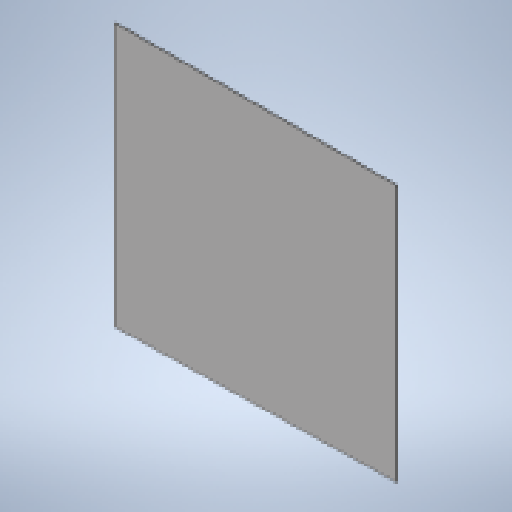
# Autodesk Inventor part: GBK 2311 shield 7
Saved by Autodesk Inventor 2026 (Build 300175000, 175)
## iProperties
Created: 2026-04-17
Part Number: GBK 2311 shield 7
Material: Steel
Document SubType Name: Sheet Metal
Designer: pokla
Stock Number: 2317
Mass: 69243.3 g
Surface Area: 44341.6 cm^2
Volume: 8820.8 cm^3
Density: 7.85 g/cm^3
Flat Pattern Width: 148 cm
Flat Pattern Length: 138.1 cm
Flat Pattern Area: 20438.8 cm^2
Sheet Metal Rule: По умолчанию_мм
Sheet Metal Width: 1480,000 мм
Sheet Metal Length: 1381,000 мм
Sheet Metal Area: 2043880,000 мм^2
Appearance: Default
Author: admin
Autodesk Inventor part; units mm, degrees
ref_plane "YZ Plane" through (0, 0, 0) normal (1, 0, 0) x (0, 1, 0)
ref_plane "XZ Plane" through (0, 0, 0) normal (0, 1, 0) x (-1, 0, 0)
ref_plane "XY Plane" through (0, 0, 0) normal (0, 0, 1) x (1, 0, 0)
sketch "Sketch1" plane through (0, 0, 0) normal (0, 0, 1) x (1, 0, 0)
  line L0 (740, -745) -> (-740, -745)
  line L1 (-740, -745) -> (-740, 745)
  line L2 (-740, 745) -> (740, 745)
  line L3 (740, 745) -> (740, -745)
  line L4 (740, -745) -> (-740, 745) construction
  line L5 (-740, -745) -> (740, 745) construction
  line L6 (-740, -636) -> (740, -602.4141)
  point P0 (0, 0)
  dimension "d0" = 1480
  dimension "d1" = 1490
  dimension "d4" = 1.3
  dimension "d9" = 1381
  dimension "d10" = 109
  measures "d0" distance of L1.end L2.end
  measures "d1" distance of L0.end L1.end
  measures "d4" angle of L0 L6
  measures "d9" distance of L1.end L6.start
  measures "d10" distance of L0.end L6.start
extrude "Plate1" add sketch "Sketch1" along normal blind 4 contours L6 L1 L2 L3
sketch "Эскиз3" plane through (0, 0, 0) normal (0, 0, -1) x (-1, 0, 0)
  line L0 (636.5062, -289.7957) -> (636.5062, -787.9319) construction
  line L1 (636.5062, -787.9319) -> (596.8789, -787.9319) construction
  line L2 (596.8789, -787.9319) -> (596.8789, -289.7957) construction
  line L3 (596.8789, -289.7957) -> (636.5062, -289.7957) construction
  line L4 (210.5058, -492.5) -> (210.5058, -589.5) projected
  line L5 (210.5058, -589.5) -> (206.5068, -589.5) projected
  line L6 (-289.6228, -492.5) -> (-289.6228, -589.5) projected
  line L7 (-289.6228, -589.5) -> (-293.6218, -589.5) projected
  ellipse E0 centre (210.5058, 745.5) end of major axis (210.5058, 775.5) minor radius 0.6803 (210.5058, 715.5) -> (210.5058, 775.5) ccw projected
  line L8 (210.5058, 715.5) -> (206.5068, 715.5) projected
  ellipse E1 centre (-289.6228, 745.5) end of major axis (-289.6228, 775.5) minor radius 0.6803 (-289.6228, 715.5) -> (-289.6228, 775.5) ccw projected
  line L9 (-289.6228, 715.5) -> (-293.6218, 715.5) projected
  line L10 (-739.3197, -489) -> (-710, -489) projected
  line L11 (-710, -489) -> (-710, -485) projected
  line L12 (-739.3197, 7.6667) -> (-710, 7.6667) projected
  line L13 (-710, 7.6667) -> (-710, 11.6667) projected
  line L14 (-739.3197, 504.3333) -> (-710, 504.3333) projected
  line L15 (-710, 504.3333) -> (-710, 508.3333) projected
  line L16 (710, -489) -> (710, -485) projected
  line L17 (710, 7.6667) -> (710, 11.6667) projected
  line L18 (710, 504.3333) -> (710, 508.3333) projected
  line L19 (710, -489) -> (680, -489)
  line L20 (710, 7.6667) -> (680, 7.6667)
  line L21 (710, 504.3333) -> (680, 504.3333)
  point P0 (0, 0)
  dimension "d14" = 30
  dimension "d15" = 30
  dimension "d16" = 30
  constraints: 6 end point, 3 horizontal, 4 other
  measures "d14" distance of L16.start L19.end
  measures "d15" distance of L17.start L20.end
  measures "d16" distance of L18.start L21.end
mark "Маркировка1"
equation "\"d0\" = Лист_ширина"
equation "\"d2\" = Thickness"
equation "\"BendRadius\" = Thickness"
equation "\"BendReliefWidth\" = Thickness"
equation "\"BendReliefDepth\" = 0.5 * Thickness"
equation "\"CornerReliefSize\" = 4 * Thickness"
equation "\"MinimumRemnant\" = 2 * Thickness"
equation "\"TransitionRadius\" = BendRadius"
equation "\"JacobiRadiusSize\" = BendRadius"
equation "\"GapSize\" = Thickness"
equation "\"Лист_ширина\" = 1480"
equation "\"Thickness\" = 4"
body "Solid1"
